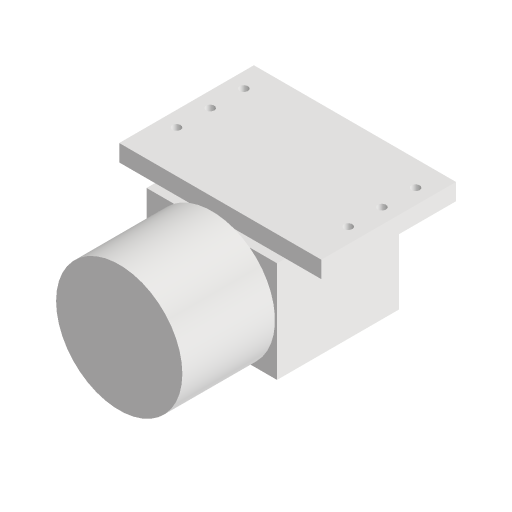
# Autodesk Inventor part: 00_Micro_Stepper_15mm_Gearbox
Saved by Autodesk Inventor 2024.1 (Build 281209000, 209)
## iProperties
Created: 2024-08-29
Part Number: 00_Micro_Stepper_15mm_Gearbox
Material: Generisch
Document SubType Name: Modeling
Designer: diederichbenedict
Density: 1 g/cm^3
Appearance: Vorgabe
Author: diederichbenedict
Autodesk Inventor part; units mm, degrees
ref_plane "YZ Plane" through (0, 0, 0) normal (1, 0, 0) x (0, 1, 0)
ref_plane "XZ Plane" through (0, 0, 0) normal (0, 1, 0) x (-1, 0, 0)
ref_plane "XY Plane" through (0, 0, 0) normal (0, 0, 1) x (1, 0, 0)
sketch "Skizze1" plane through (0, 0, 0) normal (0, 0, 1) x (1, 0, 0)
  line L0 (7.75, -7.25) -> (-7.75, -7.25)
  line L1 (-7.75, -7.25) -> (-7.75, 7.25)
  line L2 (-7.75, 7.25) -> (7.75, 7.25)
  line L3 (7.75, 7.25) -> (7.75, -7.25)
  line L4 (7.75, -7.25) -> (-7.75, 7.25) construction
  line L5 (-7.75, -7.25) -> (7.75, 7.25) construction
  point P0 (0, 0)
  dimension "d0" = 15.5
  dimension "d1" = 14.5
  constraints: 12 end point, 2 midpoint, 2 parallel, 1 horizontal, 1 perpendicular
  measures "d0" distance of L1.end L2.end
  measures "d1" distance of L0.end L1.end
extrude "Extrusion1" add sketch "Skizze1" along normal blind 12
sketch "Skizze2" plane through (0, 0, 12) normal (0, 0, 1) x (1, 0, 0)
  line L0 (12, -6.25) -> (-12, -6.25)
  line L1 (-12, -6.25) -> (-12, 9.75)
  line L2 (-12, 9.75) -> (12, 9.75)
  line L3 (12, 9.75) -> (12, -6.25)
  line L4 (12, -6.25) -> (-12, 9.75) construction
  line L5 (-12, -6.25) -> (12, 9.75) construction
  line L6 (7.75, 7.25) -> (-7.75, 7.25) projected
  point P0 (0, 0)
  point P1 (0, 1.75)
  dimension "d4" = 24
  dimension "d5" = 16
  dimension "d6" = 2.5
  constraints: 12 end point, 2 midpoint, 2 parallel, 1 horizontal, 1 perpendicular
  measures "d4" distance of L1.end L2.end
  measures "d5" distance of L0.end L1.end
  measures "d6" distance between parallel lines of L6 L2
extrude "Extrusion2" add sketch "Skizze2" along normal blind 2
sketch "Skizze3" plane through (-7.75, 7.25, 0) normal (0, 1, 0) x (1, 0, 0)
  line L0 (15.5, 0) -> (0, 0) projected
  line L1 (0, 0) -> (0, -12) projected
  line L2 (15.5, -12) -> (0, -12) projected
  line L3 (15.5, 0) -> (15.5, -12) projected
  circle A0 centre (7.75, -6) radius 1.5
  line L4 (8.8745, -5.0073) -> (8.8745, -6.9927)
  point P0 (7.75, 0)
  dimension "d9" = 3
  dimension "d10" = 1.1245
  constraints: 2 end point, 2 point on circle, 1 centre point, 1 vertical
  measures "d9" diameter of A0
  measures "d10" distance from line of L4 A0.centre
extrude "Extrusion3" add sketch "Skizze3" along normal blind 7 contours L4 A0 picked at (7.9997, -6)
sketch "Skizze4" plane through (-7.75, -7.25, 0) normal (0, -1, 0) x (1, 0, 0)
  line L0 (0, 0) -> (15.5, 0) projected
  line L1 (15.5, 0) -> (15.5, 12) projected
  line L2 (0, 12) -> (15.5, 12) projected
  line L3 (0, 0) -> (0, 12) projected
  arc A0 (8.8745, 6.9927) -> (8.8745, 5.0073) centre (7.75, 6) ccw projected
  circle A1 centre (7.75, 6) radius 7.5
  point P0 (7.75, 0)
  dimension "d13" = 15
  constraints: 1 centre point, 1 coincident
  measures "d13" diameter of A1
extrude "Extrusion4" add sketch "Skizze4" along normal blind 11 contours A1 L2 L0 | L0 A1 | A1 L2
sketch "Skizze5" plane through (0, 0, 14) normal (0, 0, 1) x (1, 0, 0)
  line L0 (12, 9.75) -> (-12, 9.75) projected
  line L1 (-12, 9.75) -> (-12, -6.25) projected
  line L2 (-12, -6.25) -> (12, -6.25) projected
  line L3 (12, -6.25) -> (12, 9.75) projected
  line L4 (-7.75, 7.25) -> (-7.75, -6.25) projected
  line L5 (7.75, -6.25) -> (7.75, 7.25) projected
  circle A0 centre (-10.2, -1.25) radius 0.5
  circle A1 centre (-10.2, 2.75) radius 0.5
  circle A2 centre (-10.2, 6.75) radius 0.5
  line L6 (0, 9.75) -> (0, -6.25)
  line L7 (12, 9.75) -> (12, -6.25)
  line L8 (7.75, 7.25) -> (7.75, -6.25)
  circle A3 centre (10.2, -1.25) radius 0.5
  circle A4 centre (10.2, 2.75) radius 0.5
  circle A5 centre (10.2, 6.75) radius 0.5
  point P0 (0, 0)
  dimension "d16" = 1
  dimension "d17" = 1
  dimension "d18" = 1
  dimension "d19" = 5
  dimension "d20" = 4
  dimension "d21" = 4
  dimension "d22" = 1.8
  dimension "d23" = 1.8
  dimension "d24" = 1.8
  constraints: 6 centre point, 6 end point, 3 symmetric about line, 2 midpoint, 3 other
  measures "d16" diameter of A0
  measures "d17" diameter of A1
  measures "d18" diameter of A2
  measures "d19" distance from line of A0.centre L2
  measures "d20" distance of A1.centre A0.centre
  measures "d21" distance of A1.centre A2.centre
  measures "d22" distance from line of L1 A2.centre
  measures "d23" distance from line of A1.centre L1
  measures "d24" distance from line of L1 A0.centre
extrude "Extrusion5" cut sketch "Skizze5" against normal blind 11 contours A0 | A1 | A2 | A3 | A4 | A5
